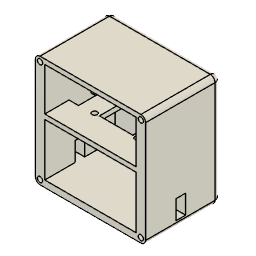
Body#2 (Autodesk Fusion 360 design; units mm, degrees)
part number: 2026-07-05-16-47-10-244
Autodesk Fusion 360 part; units mm, degrees
sketch "Sketch1" plane through (0, 0, 0) normal (0, 0, 1) x (1, 0, 0)
  line L0 (0, 0) -> (115.84, 0)
  line L1 (115.84, 0) -> (115.84, 117)
  line L2 (115.84, 117) -> (0, 117)
  line L3 (0, 117) -> (0, 0)
  line L4 (10, 7) -> (105.84, 7)
  line L5 (105.84, 7) -> (105.84, 112)
  line L6 (105.84, 112) -> (10, 112)
  line L7 (10, 112) -> (10, 7)
  line L8 (10, 67) -> (105.84, 67)
  line L9 (105.84, 67) -> (105.84, 62)
  line L10 (105.84, 62) -> (10, 62)
  line L11 (10, 62) -> (10, 67)
  circle A0 centre (5, 112) radius 2.75
  circle A1 centre (5, 5) radius 2.75
  circle A2 centre (110.84, 5) radius 2.75
  circle A3 centre (110.84, 112) radius 2.75
  circle A4 centre (5, 112) radius 1.6
  circle A5 centre (5, 5) radius 1.6
  circle A6 centre (110.84, 5) radius 1.6
  circle A7 centre (110.84, 112) radius 1.6
  dimension "d1" = 115.84
  dimension "d2" = 117
  dimension "d3" = 95.84
  dimension "d4" = 105
  dimension "d5" = 5
  dimension "d6" = 10
  dimension "d7" = 5
  dimension "d8" = 55
  dimension "d43" = 5.5
  dimension "d44" = 5
  dimension "d45" = 5
  dimension "d46" = 5.5
  dimension "d47" = 5
  dimension "d48" = 5
  dimension "d49" = 5.5
  dimension "d50" = 5
  dimension "d51" = 5
  dimension "d52" = 5.5
  dimension "d53" = 5
  dimension "d54" = 5
  dimension "d88" = 3.2
  dimension "d89" = 3.2
  dimension "d90" = 3.2
  dimension "d91" = 3.2
  constraint horizontal L0
  constraint vertical L1
  constraint horizontal L2
  constraint vertical L3
  constraint coincident L0.start L3.end
  constraint horizontal L4
  constraint vertical L5
  constraint horizontal L6
  constraint vertical L7
  constraint horizontal L8
  constraint vertical L9
  constraint horizontal L10
  constraint vertical L11
  constraint coincident L7 L8.start
  constraint concentric A0 A4
  constraint concentric A1 A5
  constraint concentric A2 A6
  constraint concentric A3 A7
  measures "d1" distance of L0.start L0.end
  measures "d2" distance of L0.start L2.end
  measures "d3" distance of L4.start L4.end
  measures "d4" distance of L4.start L6.end
  measures "d5" distance of L2 L6
  measures "d6" distance of L1 L5
  measures "d7" distance of L8.start L10.end
  measures "d8" distance of L4 L10
  measures "d43" diameter of A0
  measures "d44" distance of L3 A0.centre
  measures "d45" distance of L2 A0.centre
  measures "d46" diameter of A1
  measures "d47" distance of L0 A1.centre
  measures "d48" distance of L3 A1.centre
  measures "d49" diameter of A2
  measures "d50" distance of L1 A2.centre
  measures "d51" distance of L0 A2.centre
  measures "d52" diameter of A3
  measures "d53" distance of L1 A3.centre
  measures "d54" distance of L2 A3.centre
  measures "d88" diameter of A4
  measures "d89" diameter of A5
  measures "d90" diameter of A6
  measures "d91" diameter of A7
extrude "Extrude1" add sketch "Sketch1" against normal blind 78.85 contours L0 L1 L2 L3 | L4 L5 L7 L10 | L5 L7 L8 L9 L10 L11 | L5 L6 L7 L8 | A0 | A1 | A2 | A3 | A4 | A5 | A6 | A7
extrude "Extrude2" cut sketch "Sketch1" against normal blind 73.85 contours L4 L5 L7 L10 | L5 L6 L7 L8
extrude "Extrude7" cut sketch "Sketch1" against normal blind 5 contours A0 | A1 | A2 | A3 | A4 | A5 | A6 | A7
extrude "Extrude11" cut sketch "Sketch1" against normal blind 25 contours A4 | A5 | A6 | A7
ref_plane "WorkPlane1" through (0, 30, 0) normal (0, 1, 0) x (0, 0, 1)
sketch "Sketch2" plane through (0, 30, 0) normal (0, 1, 0) x (1, 0, 0)
  line L0 (10, 48.425) -> (20, 48.425)
  line L1 (20, 48.425) -> (20, 25.425)
  line L2 (20, 25.425) -> (10, 25.425)
  line L3 (10, 25.425) -> (10, 48.425)
  line L4 (115.84, 0) -> (0, 0)
  line L5 (105.84, 25.425) -> (90.84, 25.425)
  line L6 (90.84, 25.425) -> (90.84, 48.425)
  line L7 (90.84, 48.425) -> (105.84, 48.425)
  line L8 (105.84, 48.425) -> (105.84, 25.425)
  line L9 (0, 0) -> (0, 78.85)
  line L10 (115.84, 0) -> (115.84, 78.85)
  dimension "d14" = 10
  dimension "d15" = 23
  dimension "d16" = 25.425
  dimension "d17" = 15
  dimension "d18" = 23
  dimension "d19" = 25.425
  dimension "d20" = 10
  dimension "d21" = 10
  constraint horizontal L0
  constraint vertical L1
  constraint horizontal L2
  constraint vertical L3
  constraint horizontal L5
  constraint vertical L6
  constraint horizontal L7
  constraint vertical L8
  measures "d14" distance of L0.start L0.end
  measures "d15" distance of L0.start L2.end
  measures "d16" distance of L2 L4
  measures "d17" distance of L5.start L5.end
  measures "d18" distance of L5.start L7.end
  measures "d19" distance of L4 L5
  measures "d20" distance of L3 L9
  measures "d21" distance of L8 L10
extrude "Extrude3" cut sketch "Sketch2" along normal blind 60
ref_plane "WorkPlane2" through (125.84, 58.5, -39.425) normal (1, 0, 0) x (0, -1, 0)
sketch "Sketch3" plane through (125.84, 0, 0) normal (1, 0, 0) x (0, 0, -1)
  line L0 (31.925, 27) -> (41.925, 27)
  line L1 (41.925, 27) -> (41.925, 7)
  line L2 (41.925, 7) -> (31.925, 7)
  line L3 (31.925, 7) -> (31.925, 27)
  line L4 (0, 0) -> (78.85, 0)
  line L5 (0, 0) -> (0, 117)
  dimension "d25" = 10
  dimension "d26" = 20
  dimension "d27" = 7
  dimension "d28" = 31.925
  constraint horizontal L0
  constraint vertical L1
  constraint horizontal L2
  constraint vertical L3
  measures "d25" distance of L0.start L0.end
  measures "d26" distance of L0.start L2.end
  measures "d27" distance of L2 L4
  measures "d28" distance of L3 L5
extrude "Extrude4" cut sketch "Sketch3" against normal blind 160
fillet "Fillet1" radius 5 4 edges at (115.84, 117, -39.425) (0, 117, -39.425) (115.84, 0, -39.425) (0, 0, -39.425)
ref_plane "WorkPlane3" through (0, 70, 0) normal (0, 1, 0) x (0, 0, 1)
sketch "Sketch4" plane through (0, 70, 0) normal (0, 1, 0) x (1, 0, 0)
  line L0 (30.42, 56.925) -> (85.42, 56.925)
  line L1 (85.42, 56.925) -> (85.42, 21.925)
  line L2 (85.42, 21.925) -> (30.42, 21.925)
  line L3 (30.42, 21.925) -> (30.42, 56.925)
  line L4 (40.42, 51.925) -> (75.42, 51.925)
  line L5 (75.42, 51.925) -> (75.42, 26.925)
  line L6 (75.42, 26.925) -> (40.42, 26.925)
  line L7 (40.42, 26.925) -> (40.42, 51.925)
  circle A0 centre (35.42, 51.925) radius 2.75
  circle A1 centre (35.42, 26.925) radius 2.75
  circle A2 centre (80.42, 51.925) radius 2.75
  circle A3 centre (80.42, 26.925) radius 2.75
  line L8 (115.84, 0) -> (0, 0)
  line L9 (115.84, 0) -> (115.84, 78.85)
  circle A4 centre (35.42, 26.925) radius 1.6
  circle A5 centre (35.42, 51.925) radius 1.6
  circle A6 centre (80.42, 51.925) radius 1.6
  circle A7 centre (80.42, 26.925) radius 1.6
  dimension "d58" = 55
  dimension "d59" = 35
  dimension "d60" = 35
  dimension "d61" = 25
  dimension "d62" = 10
  dimension "d63" = 5
  dimension "d64" = 5.5
  dimension "d65" = 5
  dimension "d66" = 5
  dimension "d67" = 5.5
  dimension "d68" = 5
  dimension "d69" = 5
  dimension "d70" = 5.5
  dimension "d71" = 5
  dimension "d72" = 5
  dimension "d73" = 5.5
  dimension "d74" = 5
  dimension "d75" = 5
  dimension "d76" = 21.925
  dimension "d77" = 30.42
  dimension "d82" = 3.2
  dimension "d83" = 3.2
  dimension "d84" = 3.2
  dimension "d85" = 3.2
  constraint horizontal L0
  constraint vertical L1
  constraint horizontal L2
  constraint vertical L3
  constraint horizontal L4
  constraint vertical L5
  constraint horizontal L6
  constraint vertical L7
  constraint concentric A1 A4
  constraint concentric A0 A5
  constraint concentric A2 A6
  constraint concentric A3 A7
  measures "d58" distance of L0.start L0.end
  measures "d59" distance of L0.start L2.end
  measures "d60" distance of L4.start L4.end
  measures "d61" distance of L4.start L6.end
  measures "d62" distance of L1 L5
  measures "d63" distance of L2 L6
  measures "d64" diameter of A0
  measures "d65" distance of L3 A0.centre
  measures "d66" distance of L0 A0.centre
  measures "d67" diameter of A1
  measures "d68" distance of L2 A1.centre
  measures "d69" distance of L3 A1.centre
  measures "d70" diameter of A2
  measures "d71" distance of L1 A2.centre
  measures "d72" distance of L0 A2.centre
  measures "d73" diameter of A3
  measures "d74" distance of L1 A3.centre
  measures "d75" distance of L2 A3.centre
  measures "d76" distance of L2 L8
  measures "d77" distance of L1 L9
  measures "d82" diameter of A4
  measures "d83" diameter of A5
  measures "d84" diameter of A6
  measures "d85" diameter of A7
extrude "Extrude8" cut sketch "Sketch4" against normal blind 15 contours L4 L5 L6 L7
extrude "Extrude9" cut sketch "Sketch4" against normal blind 7 contours A0 | A1 | A2 | A3 | A4 | A5 | A6 | A7
extrude "Extrude10" cut sketch "Sketch4" against normal blind 15 contours A4 | A5 | A6 | A7
fillet "Fillet5" radius 6 8 edges at (57.92, 0, -78.85) (114.3755, 1.4645, -78.85) (115.84, 58.5, -78.85) (114.3755, 115.5355, -78.85) (57.92, 117, -78.85) (1.4645, 115.5355, -78.85) (0, 58.5, -78.85) (1.4645, 1.4645, -78.85)
